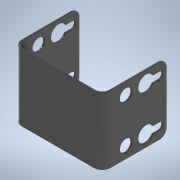
# Autodesk Inventor part: Head_back_cloth
Saved by Autodesk Inventor 2020 (Build 240168000, 168)
## iProperties
Part Number: Head_back_cloth
Material: 一般
Document SubType Name: Modeling
Designer: Masato Kubotera
Density: 1 g/cm^3
Appearance: 濃い灰色
Description: PP T0.75
Mass: 2.99646 g
Surface Area: 83.9857 cm^2
Volume: 2.99646 cm^3
Author: Masato Kubotera
Autodesk Inventor part; units mm, degrees
ref_plane "YZ Plane" through (0, 0, 0) normal (1, 0, 0) x (0, 1, 0)
ref_plane "XZ Plane" through (0, 0, 0) normal (0, 1, 0) x (-1, 0, 0)
ref_plane "XY Plane" through (0, 0, 0) normal (0, 0, 1) x (1, 0, 0)
sketch "スケッチ1" plane through (0, 0, 0) normal (1, 0, 0) x (0, 1, 0)
  line L0 (-54.6, 19) -> (54.6, 19)
  line L1 (58.6, 15) -> (58.6, -15)
  line L2 (54.6, -19) -> (-54.6, -19)
  line L3 (-58.6, -15) -> (-58.6, 15)
  line L4 (-58.6, 19) -> (58.6, -19) construction
  line L5 (58.6, 19) -> (-58.6, -19) construction
  arc A0 (-50.9799, 10.4) -> (-50.9799, 14.6) centre (-47, 12.5) ccw
  line L6 (-54.5, 10.4) -> (-50.9799, 10.4)
  line L7 (-54.5, 14.6) -> (-50.9799, 14.6)
  arc A1 (-54.5, 14.6) -> (-54.5, 10.4) centre (-54.5, 12.5) ccw
  line L8 (-54.5, 12.5) -> (-47, 12.5) construction
  line L9 (-58.6, 0) -> (58.6, 0) construction
  line L10 (-54.5, 19) -> (-54.5, -19) construction
  line L11 (-58.6, -19) -> (58.6, 19) construction
  line L12 (-54.5, -14.6) -> (-50.9799, -14.6)
  arc A2 (-54.5, -10.4) -> (-54.5, -14.6) centre (-54.5, -12.5) ccw
  line L13 (-54.5, -10.4) -> (-50.9799, -10.4)
  arc A3 (-50.9799, -14.6) -> (-50.9799, -10.4) centre (-47, -12.5) ccw
  line L14 (-54.5, -12.5) -> (-47, -12.5) construction
  line L15 (-54.5, -19) -> (-54.5, 19) construction
  line L16 (0, 19) -> (0, -19) construction
  line L17 (58.6, 19) -> (-58.6, -19) construction
  line L18 (-58.6, 19) -> (58.6, -19) construction
  line L19 (54.5, 14.6) -> (50.9799, 14.6)
  arc A4 (54.5, 10.4) -> (54.5, 14.6) centre (54.5, 12.5) ccw
  line L20 (54.5, 10.4) -> (50.9799, 10.4)
  arc A5 (50.9799, 14.6) -> (50.9799, 10.4) centre (47, 12.5) ccw
  line L21 (54.5, 12.5) -> (47, 12.5) construction
  line L22 (58.6, 0) -> (-58.6, 0) construction
  line L23 (54.5, 19) -> (54.5, -19) construction
  arc A6 (54.5, -14.6) -> (54.5, -10.4) centre (54.5, -12.5) ccw
  line L24 (54.5, -14.6) -> (50.9799, -14.6)
  line L25 (54.5, -10.4) -> (50.9799, -10.4)
  line L26 (54.5, -12.5) -> (47, -12.5) construction
  arc A7 (50.9799, -10.4) -> (50.9799, -14.6) centre (47, -12.5) ccw
  line L27 (54.5, -19) -> (54.5, 19) construction
  line L28 (58.6, -19) -> (-58.6, 19) construction
  arc A8 (-54.6, 19) -> (-58.6, 15) centre (-54.6, 15) ccw
  arc A9 (-58.6, -15) -> (-54.6, -19) centre (-54.6, -15) ccw
  arc A10 (58.6, 15) -> (54.6, 19) centre (54.6, 15) ccw
  arc A11 (54.6, -19) -> (58.6, -15) centre (54.6, -15) ccw
  line L29 (-20.5, 19) -> (-20.5, -19)
  line L30 (20.5, 19) -> (20.5, -19)
  line L31 (-16.5, 19) -> (-16.5, -19) construction
  line L32 (16.5, 19) -> (16.5, -19) construction
  line L33 (-24.5, 19) -> (-24.5, -19) construction
  line L34 (24.5, 19) -> (24.5, -19) construction
  circle A12 centre (-35.5, 12.5) radius 3.5
  circle A13 centre (-35.5, -12.5) radius 3.5
  circle A14 centre (35.5, 12.5) radius 3.5
  circle A15 centre (35.5, -12.5) radius 3.5
  point P0 (0, 0)
  point P1 (0, 0)
  point P2 (43.6458, 9.5001)
  point P3 (43.6458, 15.4999)
  point P4 (43.6458, -15.4999)
  point P5 (43.6458, -9.5001)
  point P6 (-43.6458, 15.4999)
  point P7 (-43.6458, 9.5001)
  point P8 (-43.6458, -9.5001)
  point P9 (-43.6458, -15.4999)
  dimension "d0" = 117.2
  dimension "d1" = 9
  dimension "d2" = 4.2
  dimension "d3" = 7.5
  dimension "d5" = 2
  dimension "d6" = 25
  dimension "d7" = 2
  dimension "d8" = 38
  dimension "d13" = 4
  dimension "d15" = 33
  dimension "d16" = 30
  dimension "d17" = 8
  dimension "d22" = 7
  dimension "d23" = 19
  constraints: 66 end point, 35 symmetric about line, 24 point on circle, 16 centre point, 9 point on line, 7 vertical, 6 tangent, 5 midpoint, 3 equal radius, 3 parallel, 41 other
  measures "d0" distance of L4.end L5.end
  measures "d1" diameter of A0
  measures "d2" diameter of A1
  measures "d3" distance of L8.start L8.end
  measures "d5" distance edge to line of A1 L3
  measures "d6" distance of L14.start L8.start
  measures "d8" distance of L5.start L4.end
  measures "d13" radius of A8
  measures "d15" distance of L32.start L31.start
  measures "d16" distance between parallel lines of L10 L33
  measures "d17" distance of L33.start L31.start
  measures "d22" diameter of A12
  measures "d23" distance of A12.centre L8.start
extrude "押し出し1" add sketch "スケッチ1" along normal blind 0.75
bend part "曲げパーツ1" radius 4 angle 90 line through (0, -20.5, 19) along (0, 0, -1) centre toward (-1, 0, 0) moving side (0, -1, 0) both sides no
bend part "曲げパーツ2" radius 4 angle 90 line through (0, 20.5, 19) along (0, 0, -1) centre toward (-1, 0, 0) moving side (0, 1, 0) both sides no
equation "\"d7\" = d5"
equation "\"d18\" = 0.5 * d17"
equation "\"d20\" = 0.5 * d17"
